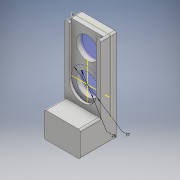
# Autodesk Inventor part: NespressoSpeedfiller
Saved by Autodesk Inventor 2017 (Build 210142000, 142)
## iProperties
Created: 2018-08-27
Part Number: NespressoSpeedfiller
Material: Generic
Document SubType Name: Modeling
Designer: 45027374
Density: 1 g/cm^3
Appearance: Default
Author: 45027374
Autodesk Inventor part; units mm, degrees
ref_plane "YZ Plane" through (0, 0, 0) normal (1, 0, 0) x (0, 1, 0)
ref_plane "XY Plane" through (0, 0, 0) normal (0, 0, 1) x (1, 0, 0)
sketch "Sketch1" plane through (0, 0, 0) normal (0, 1, 0) x (-1, 0, 0)
  line L0 (25.9, 0) -> (-25.9, 0) projected
  line L1 (0, -25.9) -> (0, 25.9) projected
  circle A0 centre (0, 0) radius 18.5 construction
  circle A1 centre (0, 0) radius 13 construction
  dimension "d0" = 37
  dimension "d1" = 26
  constraints: 2 centre point, 2 coincident
  measures "d0" diameter of A0
  measures "d1" diameter of A1
sketch "Sketch2" plane through (0, 0, 0) normal (0, 1, 0) x (-1, 0, 0)
  line L0 (29.4, 0) -> (-29.4, 0) projected
  line L1 (0, -36.8) -> (0, 73.8) projected
  line L2 (-21, 58) -> (-21, -21)
  line L3 (-21, -21) -> (21, -21)
  line L4 (21, -21) -> (21, 58)
  line L5 (-21, 58) -> (21, 58)
  point P0 (0, 0)
  dimension "d3" = 42
  dimension "d29" = 21
  dimension "d30" = 58
  constraints: 8 end point, 1 horizontal, 1 parallel, 1 other
  measures "d3" distance of L2.end L3.end
  measures "d29" distance between parallel lines of L0 L3
  measures "d30" distance between parallel lines of L5 L0
extrude "Extrusion1" add sketch "Sketch2" along normal blind 7
sketch "Sketch6" plane through (0, 0, 0) normal (0, 1, 0) x (-1, 0, 0)
  line L0 (21, -21) -> (-21, -21) projected
  line L1 (21, 58) -> (21, -21) projected
  line L2 (-21, -21) -> (21, -21)
  line L3 (21, -21) -> (21, 58)
  line L4 (-21, 58) -> (-21, -21)
  line L5 (29.4, 0) -> (-29.4, 0) projected
  line L6 (0, -36.3) -> (0, 70.8) projected
  arc A0 (-16, 0) -> (16, 0) centre (0, 0) ccw
  line L7 (16, 0) -> (16, 58)
  line L8 (21, 58) -> (-21, 58) projected
  line L9 (16, 58) -> (21, 58)
  line L10 (-16, 0) -> (-16, 58)
  line L11 (-16, 58) -> (-21, 58)
  point P0 (-17.3617, -21)
  dimension "d18" = 32
  constraints: 14 end point, 3 perpendicular, 3 point on line, 2 point on circle, 1 centre point, 1 coincident, 1 collinear, 1 horizontal, 1 parallel, 1 vertical
  measures "d18" diameter of A0
extrude "Extrusion5" add sketch "Sketch6" against normal blind 5.5 contours L0 L6 A0 L5 L1 | L0 L4 L5 A0 L6 | L5 L7 L8 L1 | L4 L8 L10 L5
sketch "Sketch4" plane through (0, 0, 0) normal (0, 0, 1) x (1, 0, 0)
  line L0 (-18.5, 0) -> (18.5, 0)
  line L1 (18.5, 0) -> (18.5, -2.5)
  line L2 (18.5, -2.5) -> (-18.5, -2.5)
  line L3 (-18.5, -2.5) -> (-18.5, 0)
  line L4 (-25.9, 0) -> (25.9, 0) projected
  line L5 (0, -3) -> (0, 0.5) projected
  point P0 (0, 0)
  dimension "d10" = 37
  dimension "d11" = 2.5
  constraints: 8 end point, 2 parallel, 1 collinear, 1 horizontal, 1 perpendicular, 1 other
  measures "d10" distance between parallel lines of L1 L3
  measures "d11" distance of L0.end L1.end
extrude "Extrusion6" cut sketch "Sketch4" against normal blind 21
sketch "Sketch5" plane through (0, 0, 0) normal (0, 1, 0) x (-1, 0, 0)
  circle A0 centre (0, 0) radius 18.5 construction
  circle A1 centre (0, 0) radius 18.5 construction
  line L0 (25.9, 0) -> (-25.9, 0) projected
  line L1 (0, -28.9) -> (0, 26.4) projected
  line L2 (-18.5, -21) -> (18.5, -21)
  line L3 (18.5, -21) -> (18.5, -18.5)
  line L4 (18.5, -18.5) -> (-18.5, -18.5)
  line L5 (-18.5, -18.5) -> (-18.5, -21)
  dimension "d25" = 37
  dimension "d26" = 21
  constraints: 8 end point, 2 parallel, 1 centre point, 1 coincident, 1 concentric, 1 horizontal, 1 perpendicular, 1 tangent, 1 other
  measures "d25" distance of L2.start L2.end
  measures "d26" distance between parallel lines of L0 L2
extrude "Extrusion7" add sketch "Sketch5" against normal blind 2.5
sketch "Sketch7" plane through (0, 0, 0) normal (0, 0, 1) x (1, 0, 0)
  line L0 (-18.5, 0) -> (18.5, 0)
  line L1 (18.5, 0) -> (18.5, -2.5)
  line L2 (18.5, -2.5) -> (-18.5, -2.5)
  line L3 (-18.5, -2.5) -> (-18.5, 0)
  line L4 (16, 0) -> (-16, 0) projected
  line L5 (-25.9, 0) -> (25.9, 0) projected
  line L6 (0, -3) -> (0, 0.5) projected
  dimension "d53" = 2.5
  dimension "d54" = 18.5
  constraints: 8 end point, 2 parallel, 1 collinear, 1 horizontal, 1 perpendicular, 1 other
  measures "d53" distance of L0.end L1.end
  measures "d54" distance between parallel lines of L6 L1
extrude "Extrusion8" cut sketch "Sketch7" along normal blind 58
sketch "Sketch8" plane through (0, 0, 0) normal (0, 1, 0) x (-1, 0, 0)
  circle A0 centre (0, 0) radius 13
  dimension "d34" = 26
  constraints: 1 centre point, 1 coincident
  measures "d34" diameter of A0
extrude "Extrusion9" cut sketch "Sketch8" along normal through all
pattern_linear "Rectangular Pattern1" count 2 spacing 37 along (0, 0, 1) of "Extrusion9"
sketch "Sketch9" plane through (0, 7, 0) normal (0, 1, 0) x (1, 0, 0)
  circle A0 centre (0, 0) radius 13
  circle A1 centre (0, 0) radius 15
  dimension "d40" = 26
  dimension "d41" = 30
  constraints: 2 centre point, 2 coincident
  measures "d40" diameter of A0
  measures "d41" diameter of A1
extrude "Extrusion10" [suppressed]
sketch "Sketch10" plane through (0, 5, 0) normal (0, 1, 0) x (1, 0, 0)
  arc A0 (16, 0) -> (-16, 0) centre (0, 0) ccw projected
  line L0 (1.5, -18) -> (-1.5, -18)
  line L1 (-29.4, 0) -> (29.4, 0) projected
  line L2 (0, 36.3) -> (0, -70.8) projected
  line L3 (1.5, -12) -> (-1.5, -12)
  line L4 (1.5, -12) -> (1.5, -18)
  line L5 (-1.5, -18) -> (-1.5, -12)
  dimension "d48" = 3
  dimension "d49" = 12
  dimension "d50" = 6
  constraints: 8 end point, 2 perpendicular, 1 horizontal, 1 parallel, 1 other
  measures "d48" distance between parallel lines of L4 L5
  measures "d49" distance between parallel lines of L1 L3
  measures "d50" distance between parallel lines of L0 L3
extrude "Extrusion11" [suppressed]
ref_plane "Work Plane1" through (0, 5, 0) normal (0, 1, 0) x (-1, 0, 0)
sketch "Sketch12" plane through (0, 5, 0) normal (0, 1, 0) x (-1, 0, 0)
  line L0 (21, 58) -> (21, -21) projected
  line L1 (21, -21) -> (-21, -21)
  line L2 (-21, -21) -> (-21, -51)
  line L3 (-21, -51) -> (21, -51)
  line L4 (21, -51) -> (21, -21)
  point P0 (0, 0)
  dimension "d61" = 42
  dimension "d62" = 30
  constraints: 8 end point, 2 parallel, 1 horizontal, 1 perpendicular
  measures "d61" distance of L2.end L3.end
  measures "d62" distance between parallel lines of L3 L1
extrude "Extrusion12" add sketch "Sketch12" against normal blind 34.5
sketch "Sketch13" plane through (0, 0, 0) normal (1, 0, 0) x (0, 1, 0)
  line L0 (-31.4, 0) -> (13.4, 0) projected
  line L1 (0, -62.5) -> (0, 32) projected
  line L2 (7, -19) -> (7, -49)
  line L3 (7, -49) -> (-25, -43.3575)
  line L4 (-25, -43.3575) -> (-25, -30.647)
  line L5 (7, -19) -> (-25, -30.647)
  point P0 (0, 0)
  dimension "d85" = 25
  dimension "d86" = 7
  dimension "d87" = 49
  dimension "d88" = 30
  dimension "d89" = 100
  dimension "d90" = 110
  constraints: 8 end point, 1 parallel, 1 vertical
  measures "d85" distance between parallel lines of L1 L4
  measures "d86" distance between parallel lines of L2 L1
  measures "d87" distance from line of L0 L2.end
  measures "d88" distance of L2.start L2.end
  measures "d89" angle of L4 L3
  measures "d90" angle of L5 L4
extrude "Extrusion14" cut sketch "Sketch13" along normal mid plane 38
sketch "Sketch14" plane through (0, 5, 0) normal (0, 1, 0) x (-1, 0, 0)
  line L0 (0, -72.3) -> (0, 76.8) projected
  line L1 (19, 56) -> (-19, 56)
  line L2 (-19, 56) -> (-19, -49)
  line L3 (-19, -49) -> (19, -49)
  line L4 (19, -49) -> (19, 56)
  line L5 (21, 58) -> (-21, 58)
  line L6 (-21, 58) -> (-21, -51)
  line L7 (-21, -51) -> (21, -51)
  line L8 (21, -51) -> (21, 58)
  line L9 (29.4, 0) -> (-29.4, 0) projected
  dimension "d91" = 51
  dimension "d92" = 58
  dimension "d93" = 42
  dimension "d94" = 38
  dimension "d95" = 56
  dimension "d96" = 49
  constraints: 16 end point, 4 parallel, 2 horizontal, 2 perpendicular, 2 other
  measures "d91" distance between parallel lines of L7 L9
  measures "d92" distance between parallel lines of L5 L9
  measures "d93" distance of L5.start L5.end
  measures "d94" distance of L1.start L1.end
  measures "d95" distance between parallel lines of L1 L9
  measures "d96" distance between parallel lines of L9 L3
extrude "Extrusion15" add sketch "Sketch14" along normal blind 8 contours L7 L6 L9 L2 L3 L0 | L0 L3 L4 L9 L8 L7 | L6 L5 L0 L1 L2 L9 | L9 L4 L1 L0 L5 L8
fillet "Fillet3" radius 2 4 edges at (21, 3.75, 58) (21, -8.25, -51) (-21, -8.25, -51) (-21, 3.75, 58)
fillet "Fillet4" radius 2 2 edges at (16, -4, 58) (-16, -4, 58)
fillet "Fillet5" radius 2 2 edges at (21, -17.5, -21) (-21, -17.5, -21)
fillet "Fillet6" radius 2 2 edges at (0, 7, 56) (0, 7, -19)
fillet "Fillet7" radius 4 2 edges at (0, -25, -30.647) (0, -25, -43.3575)
body "Solid1"
